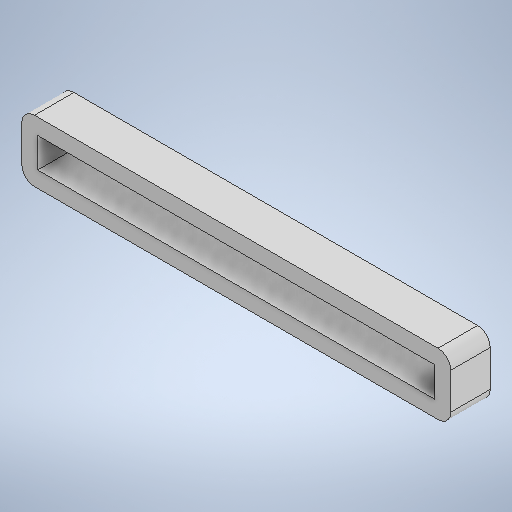
# Autodesk Inventor part: spacer
Saved by Autodesk Inventor 2025.1 (Build 291241000, 241)
## iProperties
Created: 2026-03-14
Part Number: spacer
Material: Generic
Document SubType Name: Modeling
Designer: User
Density: 1 g/cm^3
Appearance: Default
Author: User
## iProperties of the stored document spacer_3DPrint.ipt
Created: 2026-03-14
Part Number: spacer_3DPrint
Material: Generic
Document SubType Name: Modeling
Designer: User
Density: 1 g/cm^3
Appearance: Default
Author: User
Autodesk Inventor part; units mm, degrees
ref_plane "YZ Plane" through (0, 0, 0) normal (1, 0, 0) x (0, 1, 0)
ref_plane "XZ Plane" through (0, 0, 0) normal (0, 1, 0) x (-1, 0, 0)
ref_plane "XY Plane" through (0, 0, 0) normal (0, 0, 1) x (1, 0, 0)
sketch "Sketch1" plane through (0, 0, 0) normal (0, 0, 1) x (1, 0, 0)
  line L0 (30.7, 1.95) -> (-30.7, 1.95) projected
  line L1 (-30.7, 1.95) -> (-30.7, -1.75) projected
  line L2 (-30.7, 1.95) -> (30.7, 1.95)
  line L3 (30.7, 1.95) -> (30.7, -1.75)
  line L4 (30.7, -1.75) -> (-30.7, -1.75)
  line L5 (-30.7, -1.75) -> (-30.7, 1.95)
  line L6 (-31.2, -2.25) -> (31.2, -2.25)
  line L7 (31.2, -2.25) -> (31.2, 2.45)
  line L8 (31.2, 2.45) -> (-31.2, 2.45)
  line L9 (-31.2, 2.45) -> (-31.2, -2.25)
  line L10 (33.7, -4.75) -> (-33.7, -4.75)
  line L11 (-33.7, -4.75) -> (-33.7, 4.95)
  line L12 (-33.7, 4.95) -> (33.7, 4.95)
  line L13 (33.7, 4.95) -> (33.7, -4.75)
  point P0 (0, 0)
  dimension "d0" = 0.5
  dimension "d1" = 2.5
  constraints: 24 end point, 6 parallel, 3 perpendicular, 1 horizontal, 6 other
  measures "d0" distance between parallel lines of L4 L6
  measures "d1" distance between parallel lines of L6 L10
extrude "Extrusion1" add sketch "Sketch1" along normal blind 6.2 contours L10 L11 L12 L13
fillet "Fillet1" radius 2 4 edges at (33.7, -4.75, 3.1) (-33.7, -4.75, 3.1) (-33.7, 4.95, 3.1) (33.7, 4.95, 3.1)
body "Solid1"
